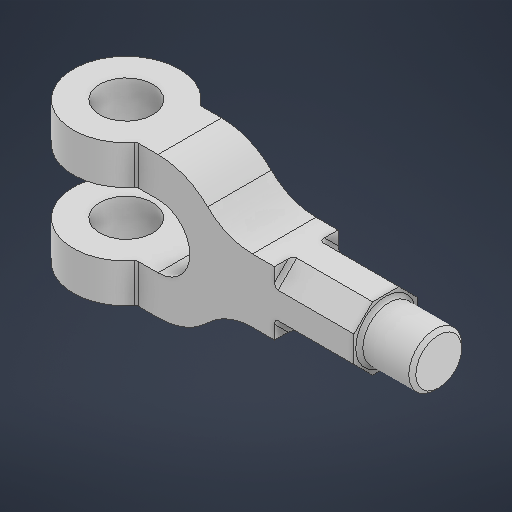
# Autodesk Inventor part: fork end
Saved by Autodesk Inventor 2026.3 (Build 303398000, 398)
## iProperties
Created: 2026-07-15
Part Number: fork end
Material: Generic
Document SubType Name: Modeling
Designer: User
Density: 1 g/cm^3
Appearance: Default
Author: User
Autodesk Inventor part; units mm, degrees
ref_plane "YZ Plane" through (0, 0, 0) normal (1, 0, 0) x (0, 1, 0)
ref_plane "XZ Plane" through (0, 0, 0) normal (0, 1, 0) x (-1, 0, 0)
ref_plane "XY Plane" through (0, 0, 0) normal (0, 0, 1) x (1, 0, 0)
sketch "Sketch2" plane through (0, 0, 0) normal (0, 0, 1) x (1, 0, 0)
  line L0 (0, 18) -> (36, 18)
  line L1 (36, -18) -> (0, -18)
  arc A0 (36, -18) -> (36, 18) centre (36, 0) ccw
  line L2 (0, 40) -> (36, 40)
  line L3 (36, -40) -> (0, -40)
  line L4 (0, 40) -> (0, 18)
  line L5 (0, -18) -> (0, -40)
  line L6 (89.479, 18) -> (147, 18)
  line L7 (147, 18) -> (147, -18)
  line L8 (147, -18) -> (89.479, -18)
  arc A1 (36, -40) -> (64.1468, -28.4211) centre (36, 0) ccw
  arc A2 (64.1468, 28.4211) -> (36, 40) centre (36, 0) ccw
  line L9 (0, 75.6) -> (0, -75.6) projected
  arc A3 (64.1468, 28.4211) -> (89.479, 18) centre (89.479, 54) ccw
  arc A4 (89.479, -18) -> (64.1468, -28.4211) centre (89.479, -54) ccw
  point P0 (0, 0)
  point P1 (0, 0)
  point P2 (71.7211, 18)
  point P3 (71.7211, -18)
  dimension "d3" = 147
  dimension "d4" = 36
  dimension "d5" = 18
  dimension "d6" = 36
  constraints: 18 end point, 12 point on circle, 5 centre point, 4 perpendicular, 4 tangent, 3 point on line, 2 parallel, 1 coincident, 1 equal radius, 1 horizontal
  measures "d3" distance between parallel lines of L7 L9
  measures "d4" radius of A3
  measures "d5" radius of A0
  measures "d6" distance of L6.end L7.end
extrude "Extrusion1" add sketch "Sketch2" along normal mid plane 36 contours L4 L2 A2 A3 L6 L7 L8 A4 A1 L3 L5 L1 A0 L0
sketch "Sketch3" plane through (0, 40, 18) normal (0, 1, 0) x (1, 0, 0)
  circle A0 centre (0, 18) radius 30
  dimension "d11" = 60
  constraints: 1 centre point, 1 coincident
  measures "d11" diameter of A0
extrude "Extrusion2" add sketch "Sketch3" against normal blind 22
sketch "Sketch4" plane through (36, 40, 18) normal (0, 1, 0) x (1, 0, 0)
  circle A0 centre (-36, 18) radius 15
  dimension "d14" = 30
  constraints: 1 centre point, 1 coincident
  measures "d14" diameter of A0
extrude "Extrusion3" cut sketch "Sketch4" against normal blind 22
mirror "Mirror1" about plane through (0, 0, 0) normal (0, 1, 0) of "Extrusion3", "Extrusion2"
sketch "Sketch5" plane through (147, -18, 18) normal (1, 0, 0) x (0, 0, -1)
  line L0 (36, 36) -> (36, 0) projected
  line L1 (36, 10.5442) -> (25.4558, 0)
  line L2 (25.4558, 0) -> (10.5442, 0)
  line L3 (10.5442, 0) -> (0, 10.5442)
  line L4 (0, 10.5442) -> (0, 25.4558)
  line L5 (0, 25.4558) -> (10.5442, 36)
  line L6 (10.5442, 36) -> (25.4558, 36)
  line L7 (25.4558, 36) -> (36, 25.4558)
  line L8 (36, 25.4558) -> (36, 10.5442)
  line L9 (36, 36) -> (0, 36) projected
  line L10 (0, 0) -> (0, 36) projected
  line L11 (36, 0) -> (0, 0) projected
  line L12 (36, 36) -> (36, 0) projected
  point P0 (18, 18)
  point P1 (18, 18)
  point P2 (36, 18)
  point P3 (36, 36)
  point P4 (36, 0)
  constraints: 16 end point, 2 midpoint, 1 coincident, 17 other
extrude "Extrusion4" cut sketch "Sketch5" against normal blind 45 contours L0 L7 L9 | L0 L11 L1 | L5 L10 L9 | L11 L10 L3
sketch "Sketch6" plane through (147, -7.4558, 18) normal (1, 0, 0) x (0, 0, -1)
  circle A0 centre (18, 7.4558) radius 15
  dimension "d19" = 30
  constraints: 1 centre point, 1 coincident
  measures "d19" diameter of A0
extrude "Extrusion5" add sketch "Sketch6" along normal blind 30
fillet "Fillet1" radius 2 9 edges at (24, 29, 18) (24, -29, 18) (102, 12.7279, 12.7279) (147, 0, 15) (24, 29, -18) (24, -29, -18) (102, 12.7279, -12.7279) (102, -12.7279, -12.7279) (102, -12.7279, 12.7279)
chamfer "Chamfer1" distance 2 angle 45 1 edges at (177, 0, 15)
body "Solid1"
